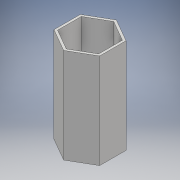
# Autodesk Inventor part: Hexagono
Saved by Autodesk Inventor 2017 (Build 210142000, 142)
## iProperties
Created: 2016-07-03
Part Number: Hexagono
Material: Generic
Document SubType Name: Modeling
Designer: Ing
Density: 1 g/cm^3
Appearance: Default
Author: Ing
Autodesk Inventor part; units mm, degrees
ref_plane "YZ Plane" through (0, 0, 0) normal (1, 0, 0) x (0, 1, 0)
ref_plane "XZ Plane" through (0, 0, 0) normal (0, 1, 0) x (-1, 0, 0)
ref_plane "XY Plane" through (0, 0, 0) normal (0, 0, 1) x (1, 0, 0)
sketch "Sketch1" plane through (0, 0, 0) normal (0, 0, 1) x (1, 0, 0)
  line L0 (0, 50) -> (43.3013, 25)
  line L1 (43.3013, 25) -> (43.3013, -25)
  line L2 (43.3013, -25) -> (0, -50)
  line L3 (0, -50) -> (-43.3013, -25)
  line L4 (-43.3013, -25) -> (-43.3013, 25)
  line L5 (-43.3013, 25) -> (0, 50)
  line L6 (0, -45) -> (-38.9711, -22.5)
  line L7 (-38.9711, -22.5) -> (-38.9711, 22.5)
  line L8 (-38.9711, 22.5) -> (0, 45)
  line L9 (0, 45) -> (38.9711, 22.5)
  line L10 (38.9711, 22.5) -> (38.9711, -22.5)
  line L11 (38.9711, -22.5) -> (0, -45)
  point P0 (0, 0)
  point P1 (0, 0)
  point P2 (0, 0)
  dimension "d0" = 50
  dimension "d2" = 5
  constraints: 24 end point, 2 coincident, 26 other
  measures "d0" distance of L3.end L4.end
  measures "d2" distance of L2.end L6.start
extrude "Extrusion1" add sketch "Sketch1" along normal blind 180
body "Solid1"
